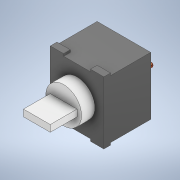
# Autodesk Inventor part: KeyboardSwitch
Saved by Autodesk Inventor 2020 (Build 240168000, 168)
## iProperties
Created: 2021-07-01
Part Number: KeyboardSwitch
Material: ABS Plastic
Document SubType Name: Modeling
Designer: 10300812
Density: 1.06 g/cm^3
Appearance: Smooth - Black
Author: 10300812
Autodesk Inventor part; units mm, degrees
ref_plane "YZ Plane" through (0, 0, 0) normal (1, 0, 0) x (0, 1, 0)
ref_plane "XZ Plane" through (0, 0, 0) normal (0, 1, 0) x (-1, 0, 0)
ref_plane "XY Plane" through (0, 0, 0) normal (0, 0, 1) x (1, 0, 0)
sketch "Sketch1" plane through (0, 0, 0) normal (0, 0, 1) x (1, 0, 0)
  line L0 (-6, 6.5) -> (6, 6.5)
  line L1 (6, 6.5) -> (6, -6.5)
  line L2 (6, -6.5) -> (-6, -6.5)
  line L3 (-6, -6.5) -> (-6, 6.5)
  line L4 (-6, 6.5) -> (6, -6.5) construction
  line L5 (6, 6.5) -> (-6, -6.5) construction
  point P0 (0, 0)
  dimension "d0" = 12
  dimension "d1" = 13
  constraints: 12 end point, 2 midpoint, 2 parallel, 1 horizontal, 1 perpendicular
  measures "d0" distance of L1.end L2.end
  measures "d1" distance of L0.end L1.end
extrude "Extrusion1" add sketch "Sketch1" along normal blind 9
sketch "Sketch2" plane through (0, 0, 9) normal (0, 0, 1) x (1, 0, 0)
  line L0 (-6, -6.5) -> (6, -6.5) projected
  line L1 (6, -6.5) -> (6, 6.5) projected
  line L2 (6, 6.5) -> (-6, 6.5) projected
  line L3 (-6, 6.5) -> (-6, -6.5) projected
  line L4 (6, 6.5) -> (-6, 6.5) projected
  line L5 (-6, 6.5) -> (-3, 6.5)
  line L6 (-3, 6.5) -> (-3, 7)
  line L7 (-3, 7) -> (-6, 7)
  line L8 (-6, 7) -> (-6, 6.5)
  line L9 (6, 6.5) -> (3, 6.5)
  line L10 (3, 6.5) -> (3, 7)
  line L11 (3, 7) -> (6, 7)
  line L12 (6, 7) -> (6, 6.5)
  line L13 (-6, -6.5) -> (6, -6.5) projected
  line L14 (6, -6.5) -> (3, -6.5)
  line L15 (3, -6.5) -> (3, -7)
  line L16 (3, -7) -> (6, -7)
  line L17 (6, -7) -> (6, -6.5)
  line L18 (-6, -6.5) -> (-3, -6.5)
  line L19 (-3, -6.5) -> (-3, -7)
  line L20 (-3, -7) -> (-6, -7)
  line L21 (-6, -7) -> (-6, -6.5)
  point P0 (0, 0)
  dimension "d4" = 3
  dimension "d5" = 0.5
  constraints: 32 end point, 8 parallel, 4 horizontal, 4 perpendicular, 3 equal length, 3 point on line
  measures "d4" distance of L6.end L7.end
  measures "d5" distance of L7.end L2.end
extrude "Extrusion2" add sketch "Sketch2" along normal blind 1.5
sketch "Sketch3" plane through (0, 0, 10.5) normal (0, 0, 1) x (1, 0, 0)
  circle A0 centre (0, 0) radius 4
  dimension "d8" = 8
  constraints: 1 centre point, 1 coincident
  measures "d8" diameter of A0
extrude "Extrusion3" add sketch "Sketch3" along normal blind 3
sketch "Sketch4" plane through (0, 0, 13.5) normal (0, 0, 1) x (1, 0, 0)
  line L0 (-3, 0.75) -> (3, 0.75)
  line L1 (3, 0.75) -> (3, -0.75)
  line L2 (3, -0.75) -> (-3, -0.75)
  line L3 (-3, -0.75) -> (-3, 0.75)
  line L4 (-3, 0.75) -> (3, -0.75) construction
  line L5 (3, 0.75) -> (-3, -0.75) construction
  point P0 (0, 0)
  dimension "d11" = 6
  dimension "d12" = 1.5
  constraints: 12 end point, 2 midpoint, 2 parallel, 1 horizontal, 1 perpendicular
  measures "d11" distance of L1.end L2.end
  measures "d12" distance of L0.end L1.end
extrude "Extrusion4" add sketch "Sketch4" along normal blind 6
sketch "Sketch5" plane through (0, 0, 0) normal (0, 0, -1) x (-1, 0, 0)
  circle A0 centre (-1.9, 0) radius 0.5
  circle A1 centre (1.9, 0) radius 0.5
  point P0 (0, 0)
  dimension "d15" = 1
  dimension "d16" = 1
  dimension "d17" = 1.9
  dimension "d18" = 1.9
  dimension "d19" = 3.8
  constraints: 2 centre point, 2 horizontal alignment
  measures "d15" diameter of A0
  measures "d16" diameter of A1
  measures "d17" distance of point (0, 0) A0.centre
  measures "d18" distance of point (0, 0) A1.centre
  measures "d19" distance of A1.centre A0.centre
extrude "Extrusion5" add sketch "Sketch5" along normal blind 4.3
fillet "Fillet1" radius 0.2 2 edges at (2.4, 0, -4.3) (-1.4, 0, -4.3)
equation "\"d18\" = d17"
body "Solid1"
